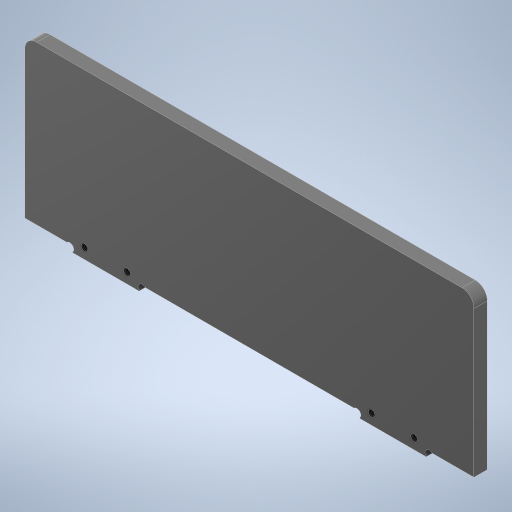
# Autodesk Inventor part: TorsoPelvisFrontCoverFrame
Saved by Autodesk Inventor 2024.2 (Build 282272000, 272)
## iProperties
Created: 2024-01-11
Part Number: TorsoPelvisFrontCoverFrame
Material: Acetal Resin, Black
Document SubType Name: Modeling
Designer: Masato Kubotera
Density: 1.425 g/cm^3
Appearance: Smooth - Black
Vendor: meviy
Mass: 22.5091 g
Surface Area: 244.77 cm^2
Volume: 15.7958 cm^3
Author: Masato Kubotera
Autodesk Inventor part; units mm, degrees
ref_plane "YZ Plane" through (0, 0, 0) normal (1, 0, 0) x (0, 1, 0)
ref_plane "XZ Plane" through (0, 0, 0) normal (0, 1, 0) x (-1, 0, 0)
ref_plane "XY Plane" through (0, 0, 0) normal (0, 0, 1) x (1, 0, 0)
sketch "Sketch1" plane through (0, 0, 0) normal (1, 0, 0) x (0, 1, 0)
  line L0 (-84.5, -30.9) -> (84.5, -30.9) construction
  line L1 (84.5, 30.9) -> (-84.5, 30.9)
  line L2 (-84.5, 30.9) -> (-84.5, -30.9) construction
  line L3 (-84.5, -30.9) -> (84.5, 30.9) construction
  line L4 (84.5, -30.9) -> (-84.5, 30.9) construction
  line L5 (-84.5, 0) -> (84.5, 0) construction
  line L6 (0, 30.9) -> (0, -30.9) construction
  line L7 (46, -27) -> (62, -27) construction
  line L8 (41.5, -30.9) -> (41.5, -23) construction
  line L9 (41.5, -23) -> (66.5, -23) construction
  line L10 (66.5, -23) -> (66.5, -30.9) construction
  line L11 (54, -23) -> (54, -30.9) construction
  line L12 (-46, -27) -> (-62, -27) construction
  line L13 (-41.5, -30.9) -> (-41.5, -23) construction
  line L14 (-41.5, -23) -> (-66.5, -23) construction
  line L15 (-66.5, -23) -> (-66.5, -30.9) construction
  line L16 (-54, -23) -> (-54, -30.9) construction
  line L17 (-84.5, 25.9) -> (69, 25.9) construction
  line L18 (41.5, -30.9) -> (41.5, -28.6)
  line L19 (41.5, -28.6) -> (-41.5, -28.6)
  line L20 (-41.5, -28.6) -> (-41.5, -30.9)
  line L21 (-66.5, -29.1) -> (66.5, -29.1) construction
  line L22 (84.5, 30.9) -> (84.5, -30.9) construction
  line L23 (66.5, -30.9) -> (66.5, -28.6)
  line L24 (66.5, -28.6) -> (84.5, -28.6)
  line L25 (-66.5, -30.9) -> (-66.5, -28.6)
  line L26 (-66.5, -28.6) -> (-84.5, -28.6)
  line L27 (82.5, 28.9) -> (82.5, 8.9)
  line L28 (82.5, -24) -> (-82.5, -24)
  line L29 (82.5, 28.9) -> (-82.5, 28.9)
  circle A0 centre (46, -27) radius 3 construction
  line L30 (82.5, 28.9) -> (82.5, -24)
  line L31 (-82.5, 28.9) -> (-82.5, -24)
  line L32 (84.5, 30.9) -> (84.5, -28.6)
  line L33 (-84.5, 30.9) -> (-84.5, -28.6)
  line L34 (66.5, -30.9) -> (41.5, -30.9)
  line L35 (-41.5, -30.9) -> (-66.5, -30.9)
  arc A1 (68.6213, -28.6) -> (66.5, -30.7213) centre (67.5607, -29.6607) ccw
  arc A2 (41.5, -30.7213) -> (39.3787, -28.6) centre (40.4393, -29.6607) ccw
  arc A3 (-66.5, -30.7213) -> (-68.6213, -28.6) centre (-67.5607, -29.6607) ccw
  arc A4 (-39.3787, -28.6) -> (-41.5, -30.7213) centre (-40.4393, -29.6607) ccw
  point P0 (0, 0)
  point P1 (-84.5, -30.9)
  point P2 (-41.5, -30.9)
  point P3 (-69, 29.5)
  point P4 (-69, 30.9)
  point P5 (-41.5, -30.9)
  point P6 (-66.5, -30.9)
  point P7 (-68.6213, -28.6)
  point P8 (-66.5, -30.7213)
  point P9 (-41.5, -30.7213)
  point P10 (-39.3787, -28.6)
  point P11 (39.3787, -28.6)
  point P12 (41.5, -30.7213)
  point P13 (-41.5, -28.6)
  point P14 (41.5, -28.6)
  point P15 (-66.5, -28.6)
  point P16 (-63.7555, -20)
  point P17 (-39.2445, -20)
  point P18 (39.2445, -20)
  point P19 (63.7555, -20)
  dimension "d0" = 169
  dimension "d2" = 16
  dimension "d3" = 3.9
  dimension "d4" = 25
  dimension "d5" = 7.9
  dimension "d18" = 5
  dimension "d35" = 2.1
  dimension "d36" = 0.5
  dimension "d38" = 108
  dimension "d47" = 2
  dimension "d50" = 6
  dimension "d53" = 2
  dimension "d56" = 1.5
  dimension "d57" = 60
  constraints: 72 end point, 27 symmetric about line, 14 point on line, 9 point on circle, 7 horizontal, 7 midpoint, 5 centre point, 5 coincident, 5 vertical, 1 collinear, 1 parallel, 1 perpendicular, 1 tangent, 1 vertical alignment, 5 other
  measures "d0" distance of L0.start L0.end
  measures "d2" distance of L7.start L7.end
  measures "d3" distance between parallel lines of L0 L7
  measures "d4" distance between parallel lines of L10 L8
  measures "d5" distance between parallel lines of L0 L9
  measures "d18" distance between parallel lines of L17 L1
  measures "d35" distance between parallel lines of L21 L7
  measures "d36" distance between parallel lines of L21 L19
  measures "d38" distance between parallel lines of L11 L16
  measures "d47" distance between parallel lines of L29 L1
  measures "d50" diameter of A0
  measures "d53" distance between parallel lines of L22 L30
  measures "d56" radius of A1
  measures "d57" distance between parallel lines of L21 L1
extrude "Extrusion1" add sketch "Sketch1" along normal blind 5 contours L32 L24 A1 L23 L34 L18 A2 L19 A4 L20 L35 L25 A3 L26 L33 L1 | L27 L30 L28 L31 L29
extrude "Extrusion2" cut sketch "Sketch1" along normal blind 4 contours L27 L30 L28 L31 L29
hole "Hole1" at (0, 46, -27) at (0, 62, -27) at (0, -62, -27) at (0, -46, -27) direction (1, 0, 0) diameter 2.459 end through all thread size "M3x0.5" class "6H" standard "ANSI Metric M Profile"
fillet "Fillet1" radius 2.5 3 edges at (2, 82.5, 28.9) (2, 82.5, -24) (2, -82.5, -24)
fillet "Fillet2" radius 2.5 1 edges at (2, -82.5, 28.9)
fillet "Fillet3" radius 4.5 2 edges at (2.5, -84.5, 30.9) (2.5, 84.5, 30.9)
equation "\"d47\" = d46"
equation "\"d46\" = 2"
body "Solid1"
